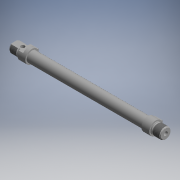
# Autodesk Inventor part: 559278 DSNU-20-200-PPS---(A----0-ZR)
Saved by Autodesk Inventor 2017.3 (Build 213256000, 256)
## iProperties
Part Number: 559278 DSNU-20-200-PPS---(A----0-ZR)
Material: Generic
Catalog Web Link: www.cadenas.de
Description: DSNU---(ZR)-Standard cylinder
Vendor: FESTO
Document SubType Name: Modeling
Designer: partserver
Manufacturer: FESTO
Mass: 45.4461 g
Surface Area: 384.345 cm^2
Volume: 45.4461 cm^3
Density: 1 g/cm^3
Appearance: PSOLRGB-192-192-192
Category: PARTsolutions
Company: FESTO
Title: 559278 DSNU-20-200-PPS
Author: Cadenas PARTsolutions
Comments: Standard cylinder
PSOL_IDENT_0: {$CADENAS_DATA\23d-libs\festo\parts\d\dsnu\parts\dsnu_metric_zr.prj},240 {VTYP=3D},{NB=559278 DSNU-2
PSOL_IDENT_1: 0-200-PPS---(A----0-ZR)},{LINA=559278 DSNU-20-200-PPS},{NN=DSNU---(ZR)},{DATE=25.01.2021 09:43:10},{
PSOL_IDENT_2: GEOMDATE=15.09.2020 12:46:13},{VERSION=},{LINEID=50},{WBVAR=TNR,HUB,DA,PE,ZD,VS,KA,K8,KP,R8},{WBNUME
PSOL_IDENT_3: RIC=HUB,K8}  {NB=559278 DSNU-20-200-PPS---(A----0-ZR)},{LINA=559278 DSNU-20-200-PPS},{KT=DUMMY},{TNR=
PSOL_IDENT_4: 559278},{TYP=DSNU-20},{DSNU=METRIC},{DE=D},{KDM=20},{HUB=200},{DA=PPS},{DA1='P','PPV','PPS'},{PE=A},
PSOL_IDENT_5: {ZD=-},{VS=-},{VSALG='-','Q'},{KA=-},{KAALG='-','S2'},{K8=0},{KP=-},{KPALG='-','KP'},{R8=-},{R81='-'
PSOL_IDENT_6: },{R8H=0.000},{A1=25},{A2=110},{A3=8},{A4=47.0},{AB=22},{AM=20},{B=22},{BB=3},{BE=M22x1,5},{BENDM=22
PSOL_IDENT_7: .000},{BEKDM=20.160},{BEP=1.500},{BS=5.5},{B1=40},{B2=0},{B3=0},{B4=0},{B5=22.4},{B6=10},{B7=0},{CD=
PSOL_IDENT_8: 8},{D=27},{D1=22},{D2=8},{D3=21.3},{D4=7.0},{D5=21.7},{D6=0},{D7=0},{EE=G1/8},{EENDM=9.7280},{EEKDM=
PSOL_IDENT_9: 8.5660},{EW=16},{F=31},{FF=M5},{FFNDM=5.000},{FFKDM=4.019},{F1=0},{H=28},{H1=0},{KK=M8},{KKNDM=8.000
PSOL_IDENT_10: 0},{KKKDM=6.4660},{KKP=0.000},{K1=M4},{K1NDM=4.000},{K1KDM=3.141},{K2=0.0},{KV=32},{KW=11},{L=12},{L
PSOL_IDENT_11: H=7.5},{LK=14.5},{L1=112},{L2=68},{L3=8.2},{L4=20.0},{L5=18},{L6=44},{L7=24},{L8=16.0},{L9=29.0},{L1
PSOL_IDENT_12: 0=82},{L11=92},{L12=66.5},{L13=116.0},{ST=5.5},{SW=7},{T=12},{WH=24},{X=2.0},{XC=95},{K1KP=36},{K2KP=
PSOL_IDENT_13: M5},{K2KPNDM=5.000},{K3KP=11},{K4KP=18.0},{K5KP=62.5},{K6KP=4.2},{K7KP=20},{K8KP=27.0},{K9KP=13.0},{
PSOL_IDENT_14: K10KP=4.5},{K11KP=20},{K12KP=M5},{K12KPNDM=5.000},{K13KP=47},{ZRSTART=36},{MHL=30.000},{ZRL=36},{C=1
PSOL_IDENT_15: 4.500},{WHX=10.000},{LD1=20.000},{LD2=19.700},{AD1=11.000},{AD2=8.000},{AD3=16.000},{AD4=8.000},{AD5=
PSOL_IDENT_16: 22.200},{MH1=9.000},{MH2=4.200},{MH3=13.000},{KP1=29.000},{KP2=14.500},{KP3=12.000},{KP4=20.000},{KP
PSOL_IDENT_17: 5=26.000},{KPC=18.000},{KPF=3.000},{KPG=17.500},{KPH=62.000},{KPJ=19.500},{KPK=17.000},{KPL=4.500},{
PSOL_IDENT_18: KPR3=1.000},{KPR=19.000},{KPS=16.000},{MLD1=35.000},{MLD2=30.000},{MLD3=4.000},{MLL1=12.000},{PPVSTD=
PSOL_IDENT_19: 12.500},{PPVMH=25.700},{PPVMQ=3.800},{PPVY=6.900},{PPVZ=8.500},{PPVA=3.900},{PPVB=0.400},{PPVC=0.600
PSOL_IDENT_20: },{PPVD=0.700},{PPVE=5.000},{PPVH=13.000},{KL1=54.3},{SWL=3.000},{K3L=4.300},{ES1=1.600},{ES2=0.000}
PSOL_IDENT_21: ,{KPVERS=0},{HUB1=200},{NUTOFF=6.500},{DIMZJREAR=308},{KAVERS=0},{VERS=1},{H2=0}
NB: 559278 DSNU-20-200-PPS---(A----0-ZR)
NN: DSNU---(ZR)
NT: Standard cylinder
NBSYN: $TNR. $TYP.-$HUB1.-$DA.---($PE.$ZD.$VS.$KA.$KP.$K8.$R8.ZR)
LINA: 559278 DSNU-20-200-PPS
CATALOG: Festo
TNR: 559278
TYP: DSNU-20
DSNU: METRIC
DE: D
KDM: 20
HUB: 200
DA: PPS
DA1: 'P','PPV','PPS'
PE: A
ZD: -
VS: -
KA: -
K8: 0
KP: -
R8: -
R81: '-'
R8H: 0
A1: 25
A2: 110
A3: 8
A4: 47
AB: 22
AM: 20
B: 22
BB: 3
BE: M22x1,5
BENDM: 22
BEKDM: 20.16
BEP: 1.5
BS: 5.5
B1: 40
B2: 0
B3: 0
B4: 0
B5: 22.4
B6: 10
B7: 0
CD: 8
D: 27
D1: 22
D2: 8
D3: 21.3
D4: 7
D5: 21.7
D6: 0
D7: 0
EE: G1/8
EENDM: 9.728
EEKDM: 8.566
EW: 16
F: 31
FF: M5
FFNDM: 5
FFKDM: 4.019
F1: 0
H: 28
H1: 0
KK: M8
KKNDM: 8
KKKDM: 6.466
KKP: 0
K1: M4
K1NDM: 4
K1KDM: 3.141
K2: 0
KV: 32
KW: 11
L: 12
LH: 7.5
LK: 14.5
L3: 8.2
L4: 20
L5: 18
L6: 44
L7: 24
L8: 16
L9: 29
L13: 116
ST: 5.5
SW: 7
T: 12
X: 2
K1KP: 36
K2KP: M5
K2KPNDM: 5
K3KP: 11
K4KP: 18
K5KP: 62.5
K6KP: 4.2
K7KP: 20
K8KP: 27
K9KP: 13
K10KP: 4.5
K11KP: 20
K12KP: M5
K12KPNDM: 5
K13KP: 47
MHL: 30
C: 14.5
WHX: 10
LD1: 20
LD2: 19.7
AD1: 11
AD2: 8
AD3: 16
AD4: 8
AD5: 22.2
MH1: 9
MH2: 4.2
MH3: 13
KP1: 29
KP2: 14.5
KP3: 12
KP4: 20
KP5: 26
KPC: 18
KPF: 3
KPG: 17.5
KPH: 62
KPJ: 19.5
KPK: 17
KPL: 4.5
KPR3: 1
KPR: 19
KPS: 16
MLD1: 35
MLD2: 30
MLD3: 4
MLL1: 12
PPVSTD: 12.5
PPVMH: 25.7
PPVMQ: 3.8
PPVY: 6.9
PPVZ: 8.5
PPVA: 3.9
PPVB: 0.4
PPVC: 0.6
PPVD: 0.7
PPVE: 5
PPVH: 13
SWL: 3
K3L: 4.3
ES1: 1.6
ES2: 0
NUTOFF: 6.5
H2: 0
SUPPLIER: FESTO
ARTICLENO: 559278 DSNU-20-200-PPS---(A----0-ZR)
BOMINFO: 559278 DSNU-20-200-PPS
CREATOR: CADENAS GmbH
Autodesk Inventor part; units mm, degrees
sketch "Sketch_1" plane through (0, 0, 0) normal (0, 0, 1) x (1, 0, 0)
  line L0 (20, 0) -> (0, 0)
  line L1 (0, 0) -> (0, 9.8)
  line L2 (0, 9.8) -> (0.2, 10)
  line L3 (0.2, 10) -> (1, 10)
  line L4 (1, 10) -> (2, 11)
  line L5 (2, 11) -> (14.95, 11)
  line L6 (14.95, 11) -> (15.8657, 10.0843)
  arc A0 (15.8657, 10.0843) -> (16.4314, 9.85) centre (16.4314, 10.65) ccw
  line L7 (16.4314, 9.85) -> (17.2, 9.85)
  arc A1 (17.2, 9.85) -> (18, 10.65) centre (17.2, 10.65) ccw
  line L8 (18, 10.65) -> (18, 11)
  line L9 (18, 11) -> (20, 11)
  line L10 (20, 11) -> (20, 0)
  line L11 (20, 0) -> (0, 0)
  constraints: 24 end point, 4 point on circle, 2 centre point
revolve "Revolution1" add sketch "Sketch_1" angle 360 about axis through (20, 0, 0) along (1, 0, 0)
thread "Thread1" size "M22x1.5" class "6g" standard "ISO Metric profile" full length
sketch "Sketch_2" plane through (20, 0, 0) normal (1, 0, 0) x (0, 0, -1)
  arc A0 (-7.3859, 11.3004) -> (7.3859, 11.3004) centre (0, 0) ccw
  arc A1 (7.25, 11.5515) -> (7.3859, 11.3004) centre (7.55, 11.5515) ccw
  line L0 (7.25, 11.5515) -> (7.25, 13.1)
  arc A2 (7.25, 13.1) -> (6.85, 13.5) centre (6.85, 13.1) ccw
  line L1 (6.85, 13.5) -> (-6.85, 13.5)
  arc A3 (-6.85, 13.5) -> (-7.25, 13.1) centre (-6.85, 13.1) ccw
  line L2 (-7.25, 13.1) -> (-7.25, 11.5515)
  arc A4 (-7.3859, 11.3004) -> (-7.25, 11.5515) centre (-7.55, 11.5515) ccw
  constraints: 10 point on circle, 6 end point, 5 centre point
extrude "Extrusion1" add sketch "Sketch_2" along normal blind 16
sketch "Sketch_3" plane through (0, 0, 0) normal (0, 0, 1) x (1, 0, 0)
  line L0 (272, 0) -> (36, 0)
  line L1 (36, 0) -> (36, 10.65)
  line L2 (36, 10.65) -> (272, 10.65)
  line L3 (272, 10.65) -> (272, 0)
  line L4 (272, 0) -> (36, 0)
  constraints: 10 end point
revolve "Revolution2" add sketch "Sketch_3" angle 360 about axis through (272, 0, 0) along (1, 0, 0)
sketch "Sketch_16" plane through (272, 0, 0) normal (1, 0, 0) x (0, 0, -1)
  arc A0 (-7.3859, 11.3004) -> (7.3859, 11.3004) centre (0, 0) ccw
  arc A1 (7.25, 11.5515) -> (7.3859, 11.3004) centre (7.55, 11.5515) ccw
  line L0 (7.25, 11.5515) -> (7.25, 13.1)
  arc A2 (7.25, 13.1) -> (6.85, 13.5) centre (6.85, 13.1) ccw
  line L1 (6.85, 13.5) -> (-6.85, 13.5)
  arc A3 (-6.85, 13.5) -> (-7.25, 13.1) centre (-6.85, 13.1) ccw
  line L2 (-7.25, 13.1) -> (-7.25, 11.5515)
  arc A4 (-7.3859, 11.3004) -> (-7.25, 11.5515) centre (-7.55, 11.5515) ccw
  constraints: 10 point on circle, 6 end point, 5 centre point
extrude "Extrusion2" add sketch "Sketch_16" along normal blind 16
sketch "Sketch_23" plane through (0, 0, 0) normal (0, 0, 1) x (1, 0, 0)
  line L0 (308, 0) -> (288, 0)
  line L1 (288, 0) -> (288, 11)
  line L2 (288, 11) -> (290, 11)
  line L3 (290, 11) -> (290, 10.65)
  arc A0 (290, 10.65) -> (290.8, 9.85) centre (290.8, 10.65) ccw
  line L4 (290.8, 9.85) -> (291.5686, 9.85)
  arc A1 (291.5686, 9.85) -> (292.1343, 10.0843) centre (291.5686, 10.65) ccw
  line L5 (292.1343, 10.0843) -> (293.05, 11)
  line L6 (293.05, 11) -> (306, 11)
  line L7 (306, 11) -> (307, 10)
  line L8 (307, 10) -> (307.8, 10)
  line L9 (307.8, 10) -> (308, 9.8)
  line L10 (308, 9.8) -> (308, 0)
  line L11 (308, 0) -> (288, 0)
  constraints: 24 end point, 4 point on circle, 2 centre point
revolve "Revolution3" add sketch "Sketch_23" angle 360 about axis through (308, 0, 0) along (1, 0, 0)
thread "Thread2" size "M22x1.5" class "6g" standard "ISO Metric profile" full length
sketch "Sketch_6" plane through (0, 0, 0) normal (0, 1, 0) x (-1, 0, 0)
  line L0 (-279, -24) -> (-279, -8)
  line L1 (-279, -8) -> (-308, -8)
  line L2 (-308, -8) -> (-308, 8)
  line L3 (-308, 8) -> (-279, 8)
  line L4 (-279, 8) -> (-279, 24)
  line L5 (-279, 24) -> (-324, 24)
  line L6 (-324, 24) -> (-324, -24)
  line L7 (-324, -24) -> (-279, -24)
  constraints: 16 end point
extrude "Extrusion3" cut sketch "Sketch_6" along normal mid plane 27
sketch "Sketch7" plane through (306, -7.5498, -8) normal (0, 0, -1) x (-1, 0, 0)
  point P0 (15, 7.5498)
hole "Hole1" at (291, 0, -8) direction (0, 0, 1) diameter 8 depth 16
sketch "Sketch8" plane through (20, 13.5, 6.85) normal (0, 1, 0) x (1, 0, 0)
  point P0 (8.2, 6.85)
hole "Hole2" at (28.2, 13.5, 0) direction (0, -1, 0) diameter 8.566 depth 13.5 countersink diameter 9.728 countersink angle 90 thread size "G9.728x0.907" designation "G 1/8" standard "ISO Pipe Threads"
sketch "Sketch9" plane through (272, 13.5, 6.85) normal (0, 1, 0) x (1, 0, 0)
  point P0 (7.8, 6.85)
hole "Hole3" at (279.8, 13.5, 0) direction (0, -1, 0) diameter 8.566 depth 16 tip angle 120 countersink diameter 9.728 countersink angle 90 thread size "G9.728x0.907" designation "G 1/8" standard "ISO Pipe Threads"
sketch "Sketch_64" plane through (0, 0, 0) normal (0, 0, 1) x (1, 0, 0)
  line L0 (255.3, 0) -> (-4, 0)
  line L1 (-4, 0) -> (-4, 4)
  line L2 (-4, 4) -> (50.3, 4)
  line L3 (50.3, 4) -> (50.3, 10)
  line L4 (50.3, 10) -> (255.3, 10)
  line L5 (255.3, 10) -> (255.3, 0)
  line L6 (255.3, 0) -> (-4, 0)
  constraints: 14 end point
revolve "Revolution4" cut sketch "Sketch_64" angle 360 about axis through (255.3, 0, 0) along (1, 0, 0)
ref_plane "FDT_FRONT_XY" through (20, 0, 0) normal (1, 0, 0) x (0, 0, -1)
ref_plane "FDT_FRONT_YZ" through (20, 0, 0) normal (0, 0, -1) x (0, 1, 0)
ref_plane "FDT_FRONT_ZX" through (20, 0, 0) normal (0, 1, 0) x (1, 0, 0)
ref_plane "FDT_QSFRONT_XY" through (28.2, 13.5, 0) normal (0, 1, 0) x (0, 0, 1)
ref_plane "FDT_QSFRONT_YZ" through (28.2, 13.5, 0) normal (0, 0, 1) x (1, 0, 0)
ref_plane "FDT_QSFRONT_ZX" through (28.2, 13.5, 0) normal (1, 0, 0) x (0, 1, 0)
ref_plane "FDT_QSREAR_XY" through (279.8, 13.5, 0) normal (0, 1, 0) x (0, 0, 1)
ref_plane "FDT_QSREAR_YZ" through (279.8, 13.5, 0) normal (0, 0, 1) x (1, 0, 0)
ref_plane "FDT_QSREAR_ZX" through (279.8, 13.5, 0) normal (1, 0, 0) x (0, 1, 0)
ref_plane "FDT_REAR_XY" through (288, 0, 0) normal (-1, 0, 0) x (0, 0, -1)
ref_plane "FDT_REAR_YZ" through (288, 0, 0) normal (0, 0, -1) x (0, -1, 0)
ref_plane "FDT_REAR_ZX" through (288, 0, 0) normal (0, -1, 0) x (-1, 0, 0)
ref_plane "FDT_SMBR1_XY" through (45.5, 0, 0) normal (-1, 0, 0) x (0, 0, 1)
ref_plane "FDT_SMBR1_YZ" through (45.5, 0, 0) normal (0, 0, 1) x (0, 1, 0)
ref_plane "FDT_SMBR1_ZX" through (45.5, 0, 0) normal (0, 1, 0) x (-1, 0, 0)
ref_plane "FDT_SMBR2_XY" through (262.5, 0, 0) normal (-1, 0, 0) x (0, 0, 1)
ref_plane "FDT_SMBR2_YZ" through (262.5, 0, 0) normal (0, 0, 1) x (0, 1, 0)
ref_plane "FDT_SMBR2_ZX" through (262.5, 0, 0) normal (0, 1, 0) x (-1, 0, 0)
ref_plane "FDT_SWIVELAXIS_XY" through (291, 0, 0) normal (0, 0, 1) x (1, 0, 0)
ref_plane "FDT_SWIVELAXIS_YZ" through (291, 0, 0) normal (1, 0, 0) x (0, 1, 0)
ref_plane "FDT_SWIVELAXIS_ZX" through (291, 0, 0) normal (0, 1, 0) x (0, 0, 1)
ref_plane "NUT_XY" through (6.5, 0, 0) normal (1, 0, 0) x (0, 0, -1)
ref_plane "NUT_YZ" through (6.5, 0, 0) normal (0, 0, -1) x (0, 1, 0)
ref_plane "NUT_ZX" through (6.5, 0, 0) normal (0, 1, 0) x (1, 0, 0)
ref_plane "ZR_XY" through (0, 0, 0) normal (1, 0, 0) x (0, 0, -1)
ref_plane "ZR_YZ" through (0, 0, 0) normal (0, 0, -1) x (0, 1, 0)
ref_plane "ZR_ZX" through (0, 0, 0) normal (0, 1, 0) x (1, 0, 0)
ref_plane "ZYL_XY" through (20, 0, 0) normal (1, 0, 0) x (0, 0, -1)
ref_plane "ZYL_YZ" through (20, 0, 0) normal (0, 0, -1) x (0, 1, 0)
ref_plane "ZYL_ZX" through (20, 0, 0) normal (0, 1, 0) x (1, 0, 0)
body "Solid1"
